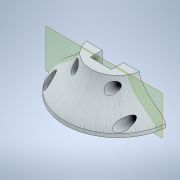
# Autodesk Inventor part: Podstawa 01-1
Saved by Autodesk Inventor 2021 (Build 250183000, 183)
## iProperties
Created: 2021-11-03
Part Number: Podstawa 01-1
Material: Generic
Document SubType Name: Modeling
Designer: Łukasz
Density: 1 g/cm^3
Appearance: Wood - Painted White
Author: Łukasz
Autodesk Inventor part; units mm, degrees
ref_plane "YZ Plane" through (0, 0, 0) normal (1, 0, 0) x (0, 1, 0)
ref_plane "XZ Plane" through (0, 0, 0) normal (0, 1, 0) x (-1, 0, 0)
ref_plane "XY Plane" through (0, 0, 0) normal (0, 0, 1) x (1, 0, 0)
sketch "Sketch1" plane through (0, 0, 0) normal (0, 0, 1) x (1, 0, 0)
  line L0 (0, 0) -> (-75, 0)
  line L1 (0, 0) -> (0, 50)
  line L2 (0, 50) -> (-38, 50)
  line L3 (-75, 0) -> (-75, 5)
  spline S0 degree 3 poles (-38, 50) (-46.7224, 6.6996) (-125.1064, 18.5226) (-28.5296, -55.0422) knots 0 0 0 0 1 1 1 1
  point P0 (-58.1914, 22.009)
  dimension "d0" = 75
  dimension "d1" = 50
  dimension "d2" = 38
  dimension "d3" = 5
  constraints: 8 end point, 2 horizontal, 2 vertical, 4 other
  measures "d0" distance of L0.start L0.end
  measures "d1" distance of L0.start L1.end
  measures "d2" distance of L1.end L2.end
  measures "d3" distance of L0.end L3.end
revolve "Revolution1" add sketch "Sketch1" angle 360 about axis through (0, 0, 0) along (0, 1, 0)
sketch "Sketch2" plane through (0, 50, 0) normal (0, 1, 0) x (1, 0, 0)
  line L0 (-15, 24) -> (15, 24)
  line L1 (15, 24) -> (15, -24)
  line L2 (15, -24) -> (-15, -24)
  line L3 (-15, -24) -> (-15, 24)
  point P0 (0, 0)
  dimension "d5" = 30
  dimension "d6" = 48
  dimension "d7" = 24
  dimension "d8" = 15
  constraints: 8 end point, 2 parallel, 1 horizontal, 1 perpendicular
  measures "d5" distance of L1.end L2.end
  measures "d6" distance of L0.end L1.end
  measures "d7" distance from line of point (0, 0) L0
  measures "d8" distance from line of L3 point (0, 0)
extrude "Extrusion1" cut sketch "Sketch2" against normal blind 35
sketch "Sketch3" plane through (0, 15, 0) normal (0, 1, 0) x (1, 0, 0)
  line L0 (15, -24) -> (-15, -24) projected
  line L1 (-15, -24) -> (-15, 24) projected
  line L2 (15, -24) -> (-15, -24)
  line L3 (-15, -24) -> (-15, -7)
  line L4 (-15, -7) -> (15, -7)
  line L5 (15, -7) -> (15, -24)
  point P0 (0, 0)
  dimension "d11" = 17
  constraints: 8 end point, 2 parallel, 1 horizontal, 1 perpendicular, 1 point on line
  measures "d11" distance of L2.end L3.end
extrude "Extrusion2" cut sketch "Sketch3" against normal blind 8
sketch "Sketch4" plane through (0, 0, 0) normal (0, 0, 1) x (1, 0, 0)
  circle A0 centre (-26, 38) radius 2.6
  circle A1 centre (-53, 12) radius 2.6
  line L0 (75, 0) -> (-75, 0) projected
  line L1 (38, 50) -> (-38, 50) projected
  line L2 (-75, 0) -> (-75, 5) projected
  line L3 (15, 50) -> (-15, 50) construction
  line L4 (0, 50) -> (0, 20.8019) construction
  circle A2 centre (26, 38) radius 2.6
  circle A3 centre (53, 12) radius 2.6
  point P0 (0, 0)
  dimension "d14" = 5.2
  dimension "d15" = 5.2
  dimension "d16" = 12
  dimension "d17" = 12
  dimension "d18" = 22
  dimension "d19" = 12
  constraints: 4 centre point, 2 end point, 2 symmetric about line, 1 midpoint, 1 vertical, 2 other
  measures "d14" diameter of A0
  measures "d15" diameter of A1
  measures "d16" distance from line of L0 A1.centre
  measures "d17" distance from line of L1 A0.centre
  measures "d18" distance from line of L2 A1.centre
  measures "d19" horizontal distance of L1.end A0.centre
extrude "Extrusion3" cut sketch "Sketch4" along normal blind 52 and the other way blind 52
ref_plane "Work Plane1" through (-15, 15, 7) normal (0, 0, 1) x (1, 0, 0)
split "Split1" plane through (-15, 15, 7) removes the side toward (0, 0, -1)
sketch "Sketch6" plane through (0, 0, 0) normal (0, -1, 0) x (1, 0, 0)
  circle A0 centre (0, 0) radius 10.5
  dimension "d25" = 21
  constraints: 1 centre point, 1 coincident
  measures "d25" diameter of A0
extrude "Extrusion4" cut sketch "Sketch6" against normal blind 2.5
ref_plane "Work Plane2" through (15, 7, 19.5) normal (0, 0, -1) x (-1, 0, 0)
sketch "Sketch7" plane through (15, 7, 19.5) normal (0, 0, -1) x (-1, 0, 0)
  circle A0 centre (41, 31) radius 2.6 projected
  circle A1 centre (41, 31) radius 6.25
  circle A2 centre (-11, 31) radius 2.6 projected
  circle A3 centre (-11, 31) radius 6.25
  circle A4 centre (-38, 5) radius 2.6 projected
  circle A5 centre (-38, 5) radius 6.25
  circle A6 centre (68, 5) radius 2.6 projected
  circle A7 centre (68, 5) radius 6.25
  point P0 (15, -7)
  dimension "d29" = 12.5
  dimension "d30" = 12.5
  dimension "d31" = 12.5
  dimension "d32" = 12.5
  constraints: 4 centre point, 4 coincident
  measures "d29" diameter of A1
  measures "d30" diameter of A3
  measures "d31" diameter of A5
  measures "d32" diameter of A7
extrude "Extrusion5" cut sketch "Sketch7" against normal blind 50 contours A0 | A1 | A2 | A3 | A4 | A5 | A6 | A7
equation "\"d7\" = 0.5 * d6"
equation "\"d8\" = 0.5 * d5"
body "Solid1"
